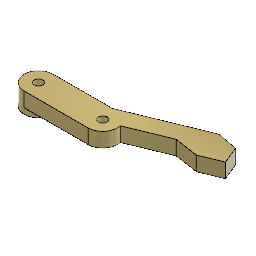
Garra_1.b_v6 (Autodesk Fusion 360 design; units mm, degrees)
Autodesk Fusion 360 part; units mm, degrees
sketch "Sketch1" plane through (0, 0, 0) normal (0, 1, 0) x (1, 0, 0)
  line L0 (0, -5) -> (22, -5)
  arc A0 (22, -5) -> (22, 5) centre (22, 0) ccw
  line L1 (22, 5) -> (0, 5)
  arc A1 (0, 5) -> (0, -5) centre (0, 0) ccw
  line L2 (0, 0) -> (22, 0) construction
  circle A2 centre (0, 0) radius 1.5
  line L3 (20.35, 5) -> (51.8071, 17.9015)
  line L4 (51.8071, 17.9015) -> (55.6974, 8.4161)
  line L5 (55.6974, 8.4161) -> (23.8973, -4.626)
  line L6 (46.255, 15.6244) -> (53.278, 14.3153)
  line L7 (48.6059, 5.5077) -> (40.4462, 6.7233)
  line L8 (40.4462, 6.7233) -> (26.8652, 1.1533)
  circle A3 centre (22, 0) radius 1.5
  dimension "d1" = 22
  dimension "d3" = 5
  dimension "d4" = 3
  dimension "d5" = 157.7
  dimension "d6" = 34
  dimension "d7" = 1.65
  dimension "d8" = 3
  constraint tangent L0 A0
  constraint tangent A0 L1
  constraint parallel L0 L1
  constraint tangent L1 A1
  constraint tangent L0 A1
  constraint horizontal L2
  constraint coincident A1.centre L2.start
  constraint coincident L1 L3.start
  constraint perpendicular L3 L4
  constraint coincident A0 L5.end
  constraint tangent A0 L5
  constraint perpendicular L4 L5
  constraint coincident L3 L6.start
  constraint coincident L4 L6.end
  constraint coincident L5 L7.start
  constraint coincident A0 L8.end
  constraint parallel L5 L8
  constraint concentric A0 A3
  measures "d1" distance of A1.centre A0.centre
  measures "d3" radius of A1
  measures "d4" diameter of A2
  measures "d5" angle of L1 L3
  measures "d6" distance of L3.start L3.end
  measures "d7" horizontal distance of A0.centre L3.start
  measures "d8" diameter of A3
extrude "Extrude1" add sketch "Sketch1" along normal blind 5 contours L0 A0 L1 A1 | A0 L1 L3 L4 L5 L6 L7 L8
sketch "Sketch2" plane through (0, 0, 0) normal (0, 1, 0) x (1, 0, 0)
sketch "Sketch4" plane through (0, 0, 0) normal (0, -1, 0) x (1, 0, 0)
  circle A0 centre (0, 0) radius 1.5
  circle A1 centre (22, 0) radius 1.5
  line L0 (0, -5) -> (20.35, -5)
  line L1 (20.35, -5) -> (46.255, -15.6244)
  line L2 (46.255, -15.6244) -> (53.278, -14.3153)
  line L3 (53.278, -14.3153) -> (55.6974, -8.4161)
  line L4 (55.6974, -8.4161) -> (48.6059, -5.5077)
  line L5 (48.6059, -5.5077) -> (40.4462, -6.7233)
  line L6 (40.4462, -6.7233) -> (26.8652, -1.1533)
  arc A2 (26.8652, -1.1533) -> (22, 5) centre (22, 0) ccw
  line L7 (22, 5) -> (0, 5)
  arc A3 (0, 5) -> (0, -5) centre (0, 0) ccw
  circle A4 centre (0, 0) radius 5
  dimension "d14" = 10
  constraint concentric A0 A4
  measures "d14" diameter of A4
extrude "Extrude3" add sketch "Sketch4" along normal blind 2 contours A3 A4
